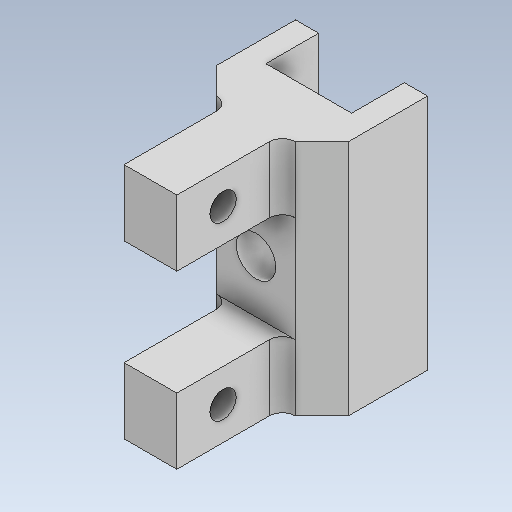
# Autodesk Inventor part: bbearing_holder_1
Saved by Autodesk Inventor 2020 (Build 240168000, 168)
## iProperties
Created: 2020-01-21
Part Number: bbearing_holder_1
Material: Generic
Document SubType Name: Modeling
Designer: psrobotics
Density: 1 g/cm^3
Appearance: Default
Author: psrobotics
Autodesk Inventor part; units mm, degrees
ref_plane "YZ Plane" through (0, 0, 0) normal (1, 0, 0) x (0, 1, 0)
ref_plane "XZ Plane" through (0, 0, 0) normal (0, 1, 0) x (-1, 0, 0)
ref_plane "XY Plane" through (0, 0, 0) normal (0, 0, 1) x (1, 0, 0)
sketch "Sketch1" plane through (0, 0, 0) normal (0, 0, 1) x (1, 0, 0)
  circle A0 centre (0, 0) radius 1.5 projected
  line L0 (-3.25, 2.3318) -> (-3.25, -2.3318) projected
  arc A1 (-3.25, -2.3318) -> (3.25, -2.3318) centre (0, 0) ccw projected
  line L1 (3.25, -2.3318) -> (3.25, 2.3318) projected
  arc A2 (3.25, 2.3318) -> (-3.25, 2.3318) centre (0, 0) ccw projected
  line L2 (5, 4) -> (5, -4)
  line L3 (5, -4) -> (-5, -4)
  line L4 (-5, -4) -> (-5, 4)
  line L5 (-5, 4) -> (5, 4)
  line L6 (5, 4) -> (-5, -4) construction
  line L7 (5, -4) -> (-5, 4) construction
  dimension "d0" = 8
  dimension "d1" = 10
  constraints: 12 end point, 3 parallel, 2 midpoint, 1 perpendicular
  measures "d0" distance of L2.start L2.end
  measures "d1" distance of L2.end L3.end
extrude "Extrusion1" add sketch "Sketch1" along normal blind 4 contours A0 | A2 L1 A1 L0 | L0 A1 L3 L4 L5 A2 | L5 L2 L3 A1 L1 A2
sketch "Sketch2" plane through (0, 0, 4) normal (0, 0, 1) x (1, 0, 0)
  line L0 (5, 4) -> (-5, 4) projected
  line L1 (-5, 4) -> (-5, -4) projected
  line L2 (-5, -4) -> (5, -4) projected
  line L3 (5, -4) -> (5, 4) projected
  circle A0 centre (0, 0) radius 1.5
  dimension "d4" = 3
  constraints: 1 centre point, 1 coincident
  measures "d4" diameter of A0
extrude "Extrusion2" cut sketch "Sketch2" against normal blind 4 contours A0
sketch "Sketch3" plane through (0, 0, 0) normal (0, 0, -1) x (-1, 0, 0)
  circle A0 centre (0, 0) radius 1.5 projected
  line L0 (-5, 4) -> (5, 4) projected
  line L1 (-5, -4) -> (-5, 4) projected
  line L2 (5, -4) -> (-5, -4) projected
  line L3 (5, 4) -> (5, -4) projected
  line L4 (-3.25, -2.3318) -> (-3.25, 2.3318) projected
  line L5 (3.25, 2.3318) -> (3.25, -2.3318) projected
  line L6 (-5, -4) -> (-3.25, -4)
  line L7 (-3.25, -4) -> (-3.25, 4)
  line L8 (-3.25, 4) -> (-5, 4)
  line L9 (-5, 4) -> (-5, -4)
  line L10 (5, 4) -> (5, -4) projected
  line L11 (5, -4) -> (3.25, -4)
  line L12 (3.25, -4) -> (3.25, 4)
  line L13 (3.25, 4) -> (5, 4)
  line L14 (5, 4) -> (5, -4)
  dimension "d7" = 1.75
  dimension "d8" = 8
  dimension "d9" = 1.75
  dimension "d10" = 8
  constraints: 16 end point, 4 parallel, 2 horizontal, 2 perpendicular
  measures "d7" distance of L8.end L7.end
  measures "d8" distance of L7.end L6.end
  measures "d9" distance of L12.end L13.end
  measures "d10" distance of L11.end L12.end
extrude "Extrusion3" add sketch "Sketch3" along normal blind 4 contours L0 L7 L4 L2 L1 | L0 L3 L2 L12 L5
sketch "Sketch4" plane through (0, 0, 4) normal (0, 0, 1) x (1, 0, 0)
  circle A0 centre (0, 0) radius 1.5 projected
  line L0 (5, 4) -> (-5, 4) projected
  line L1 (-5, 4) -> (-5, -4) projected
  line L2 (-5, -4) -> (5, -4) projected
  line L3 (5, -4) -> (5, 4) projected
  line L4 (5, -4) -> (-5, -4)
  line L5 (-5, -4) -> (-5, -9)
  line L6 (-5, -9) -> (5, -9)
  line L7 (5, -9) -> (5, -4)
  line L8 (5, -4) -> (5, 4) projected
  line L9 (5, 4) -> (-5, 4)
  line L10 (-5, 4) -> (-5, 9)
  line L11 (-5, 9) -> (5, 9)
  line L12 (5, 9) -> (5, 4)
  dimension "d13" = 10
  dimension "d14" = 5
  dimension "d15" = 10
  dimension "d16" = 5
  constraints: 16 end point, 4 parallel, 2 horizontal, 2 perpendicular
  measures "d13" distance of L6.end L5.end
  measures "d14" distance of L5.end L4.end
  measures "d15" distance of L10.end L11.end
  measures "d16" distance of L9.end L10.end
extrude "Extrusion4" add sketch "Sketch4" along normal blind 8 contours L0 L10 L11 L12 | L7 L6 L5 L2
sketch "Sketch5" plane through (-3.25, -4, 0) normal (0, -1, 0) x (1, 0, 0)
  line L0 (0, 0) -> (6.5, 0) projected
  line L1 (6.5, 0) -> (6.5, -4) projected
  line L2 (8.25, -4) -> (6.5, -4) projected
  line L3 (8.25, -4) -> (8.25, 4) projected
  line L4 (-1.75, 4) -> (8.25, 4) projected
  line L5 (-1.75, -4) -> (-1.75, 4) projected
  line L6 (0, -4) -> (-1.75, -4) projected
  line L7 (0, 0) -> (0, -4) projected
  point P0 (3.25, 0)
extrude "Extrusion5" add sketch "Sketch5" along normal up to surface (5 mm away)
sketch "Sketch6" plane through (-3.25, 4, 0) normal (0, 1, 0) x (1, 0, 0)
  line L0 (6.5, 0) -> (0, 0) projected
  line L1 (0, 0) -> (0, 4) projected
  line L2 (-1.75, 4) -> (0, 4) projected
  line L3 (-1.75, 4) -> (-1.75, -4) projected
  line L4 (8.25, -4) -> (-1.75, -4) projected
  line L5 (8.25, -4) -> (8.25, 4) projected
  line L6 (6.5, 4) -> (8.25, 4) projected
  line L7 (6.5, 0) -> (6.5, 4) projected
  point P0 (3.25, 0)
extrude "Extrusion6" add sketch "Sketch6" along normal up to surface (5 mm away)
sketch "Sketch7" plane through (5, -9, -4) normal (1, 0, 0) x (0, 0, -1)
  line L0 (-8, 5) -> (-8, 13) projected
  line L1 (-8, 5) -> (-16, 5) projected
  line L2 (-16, 0) -> (-16, 5) projected
  line L3 (0, 0) -> (-16, 0) projected
  line L4 (0, 0) -> (0, 18) projected
  line L5 (0, 18) -> (-16, 18) projected
  line L6 (-16, 13) -> (-16, 18) projected
  line L7 (-8, 13) -> (-16, 13) projected
  line L8 (-8, 5) -> (-16, 5) projected
  line L9 (0, 0) -> (-16, 0) projected
  line L10 (-8, 5) -> (-16, 5)
  line L11 (-16, 5) -> (-16, 0)
  line L12 (-16, 0) -> (-8, 0)
  line L13 (-8, 0) -> (-8, 5)
  line L14 (-16, 18) -> (-16, 13) projected
  line L15 (-8, 13) -> (-16, 13)
  line L16 (-16, 13) -> (-16, 18)
  line L17 (-16, 18) -> (-8, 18)
  line L18 (-8, 18) -> (-8, 13)
  point P0 (-4, 9)
  point P1 (-8, 18)
  point P2 (-8, 0)
  constraints: 16 end point, 4 parallel, 2 horizontal, 2 perpendicular
extrude "Extrusion7" cut sketch "Sketch7" against normal blind 3 contours L13 L3 L2 L1 | L7 L6 L5 L18
sketch "Sketch8" plane through (-5, -9, -4) normal (-1, 0, 0) x (0, 0, 1)
  line L0 (8, 18) -> (8, 13) projected
  line L1 (8, 5) -> (8, 0) projected
  line L2 (8, 13) -> (8, 5) projected
  line L3 (8, 13) -> (16, 13) projected
  line L4 (16, 18) -> (16, 13) projected
  line L5 (16, 18) -> (0, 18) projected
  line L6 (0, 18) -> (0, 0) projected
  line L7 (0, 0) -> (16, 0) projected
  line L8 (16, 5) -> (16, 0) projected
  line L9 (8, 5) -> (16, 5) projected
  point P0 (4, 9)
extrude "Extrusion8" cut sketch "Sketch8" against normal blind 3 contours L5 L4 L3 L0 | L9 L8 L7 L1
sketch "Sketch9" plane through (2, -9, -4) normal (1, 0, 0) x (0, 0, -1)
  line L0 (-8, 13) -> (-16, 13) projected
  line L1 (-8, 18) -> (-8, 13) projected
  line L2 (-16, 18) -> (-8, 18) projected
  line L3 (-16, 13) -> (-16, 18) projected
  line L4 (-16, 0) -> (-16, 5) projected
  line L5 (-8, 0) -> (-16, 0) projected
  line L6 (-8, 5) -> (-8, 0) projected
  line L7 (-16, 5) -> (-8, 5) projected
  line L8 (-16, 13) -> (-16, 18) projected
  line L9 (-16, 15.5) -> (-12.5, 15.5)
  circle A0 centre (-12.5, 15.5) radius 1
  line L10 (-16, 2.5) -> (-12.5, 2.5)
  circle A1 centre (-12.5, 2.5) radius 1
  point P0 (-4, 9)
  dimension "d27" = 3.5
  dimension "d28" = 2
  dimension "d29" = 3.5
  dimension "d30" = 2
  constraints: 4 end point, 2 centre point, 2 coincident, 2 horizontal, 2 midpoint
  measures "d27" distance of L9.start L9.end
  measures "d28" diameter of A0
  measures "d29" distance of L10.start L10.end
  measures "d30" diameter of A1
extrude "Extrusion9" cut sketch "Sketch9" against normal blind 4 contours A0 | A1
chamfer "Chamfer1" distance 2 angle 45 2 edges at (5, 0, 4) (-5, 0, 4)
fillet "Fillet1" radius 1 4 edges at (2, 6.5, 4) (2, -6.5, 4) (-2, -6.5, 4) (-2, 6.5, 4)
body "Solid1"
